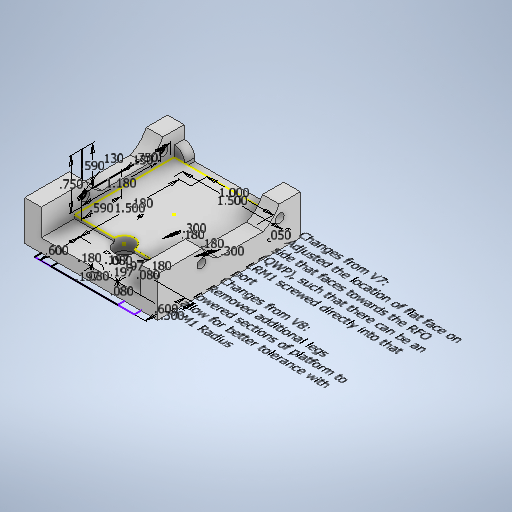
# Autodesk Inventor part: BeamsplitterMounttoPolarisPinAdapterV9
Saved by Autodesk Inventor 2025.2 (Build 292293000, 293)
## iProperties
Created: 2024-02-07
Part Number: BeamsplitterMounttoPolarisPinAdapterV9
Material: Generic
Document SubType Name: Modeling
Designer: monolithic
Density: 1 g/cm^3
Appearance: Default
Author: monolithic
Autodesk Inventor part; units mm, degrees
ref_plane "YZ Plane" through (0, 0, 0) normal (1, 0, 0) x (0, 1, 0)
ref_plane "XZ Plane" through (0, 0, 0) normal (0, 1, 0) x (-1, 0, 0)
ref_plane "XY Plane" through (0, 0, 0) normal (0, 0, 1) x (1, 0, 0)
sketch "Sketch1" plane through (0, 0, 0) normal (0, 1, 0) x (-1, 0, 0)
  line L0 (-12.7, 19.05) -> (12.7, 19.05)
  line L1 (12.7, 19.05) -> (12.7, -19.05)
  line L2 (12.7, -19.05) -> (-12.7, -19.05)
  line L3 (-12.7, -19.05) -> (-12.7, 19.05)
  line L4 (-12.7, 19.05) -> (12.7, -19.05) construction
  line L5 (12.7, 19.05) -> (-12.7, -19.05) construction
  circle A0 centre (0, 0) radius 2.286
  line L6 (12.7, 19.05) -> (-12.7, 19.05)
  line L7 (-12.7, 19.05) -> (-12.7, 34.29)
  line L8 (-12.7, 34.29) -> (12.7, 34.29)
  line L9 (12.7, 34.29) -> (12.7, 19.05)
  line L10 (-19.05, 19.05) -> (19.05, 19.05)
  line L11 (19.05, 19.05) -> (19.05, -19.05)
  line L12 (19.05, -19.05) -> (-19.05, -19.05)
  line L13 (-19.05, -19.05) -> (-19.05, 19.05)
  line L14 (-19.05, 19.05) -> (19.05, -19.05) construction
  line L15 (19.05, 19.05) -> (-19.05, -19.05) construction
  circle A1 centre (12.7, 0) radius 2.286
  circle A2 centre (-12.7, 0) radius 2.286
  line L16 (19.05, 19.05) -> (-19.05, 19.05)
  line L17 (-19.05, 19.05) -> (-19.05, 34.29)
  line L18 (-19.05, 34.29) -> (19.05, 34.29)
  line L19 (19.05, 34.29) -> (19.05, 19.05)
  circle A3 centre (0, 26.67) radius 2.286
  line L20 (-19.05, -19.05) -> (19.05, -19.05)
  line L21 (19.05, -19.05) -> (19.05, -20.32)
  line L22 (19.05, -20.32) -> (-19.05, -20.32)
  line L23 (-19.05, -20.32) -> (-19.05, -19.05)
  circle A4 centre (0, 0) radius 3.81
  circle A5 centre (-12.7, 0) radius 3.81
  circle A6 centre (12.7, 0) radius 3.81
  line L24 (0, 26.67) -> (-5.0038, 26.67)
  line L25 (-5.0038, 26.67) -> (0, 26.67)
  line L26 (0, 26.67) -> (5.0038, 26.67)
  circle A7 centre (5.0038, 26.67) radius 1.016
  circle A8 centre (-5.0038, 26.67) radius 1.016
  circle A9 centre (0, 19.05) radius 2.286
  line L27 (-19.05, 26.67) -> (19.05, 26.67)
  line L28 (0, 19.05) -> (5.004, 19.05)
  line L29 (0, 19.05) -> (-5.004, 19.05)
  circle A10 centre (5.004, 19.05) radius 1.016
  circle A11 centre (-5.004, 19.05) radius 1.016
  point P0 (12.7, 34.29)
  dimension "d0" = 38.1
  dimension "d1" = 25.4
  dimension "d2" = 4.572
  dimension "d3" = 15.24
  dimension "d4" = 38.1
  dimension "d5" = 4.572
  dimension "d6" = 4.572
  dimension "d7" = 4.572
  dimension "d10" = 1.27
  dimension "d13" = 15.24
  dimension "d14" = 7.62
  dimension "d15" = 7.62
  dimension "d16" = 7.62
  dimension "d22" = 5.0038
  dimension "d23" = 5.0038
  dimension "d24" = 2.032
  dimension "d25" = 2.032
  dimension "d28" = 4.572
  dimension "d74" = 5.004
  dimension "d75" = 5.004
  dimension "d76" = 2.032
  dimension "d77" = 2.032
  constraints: 60 end point, 12 centre point, 11 equal length, 9 coincident, 9 midpoint, 6 horizontal, 5 perpendicular, 3 point on line
  measures "d0" distance of L0.end L1.end
  measures "d1" distance of L1.end L2.end
  measures "d2" diameter of A0
  measures "d3" distance of L8.end L0.end
  measures "d4" distance of L11.end L12.end
  measures "d5" diameter of A1
  measures "d6" diameter of A2
  measures "d7" diameter of A3
  measures "d10" distance of L22.end L12.end
  measures "d13" distance of L16.end L17.end
  measures "d14" distance of point (0, 19.05) L24.start
  measures "d15" diameter of A4
  measures "d16" diameter of A5
  measures "d22" distance of L24.start L24.end
  measures "d23" distance of L24.start L26.end
  measures "d24" diameter of A7
  measures "d25" diameter of A8
  measures "d28" diameter of A9
  measures "d74" distance of L28.start L28.end
  measures "d75" distance of L28.start L29.end
  measures "d76" diameter of A10
  measures "d77" diameter of A11
extrude "Extrusion1" add sketch "Sketch1" along normal blind 6.35 contours L0 A11 | L0 A11 | A11 L0 L7 L27 A8 L24 A3 L26 A7 L9 A10 A9 | L0 A9 A10 L1 A6 L2 L3 A5 A11 | L10 L17 L27 L7 | L3 A5 L12 L13 L10 | A5 L3 A2 | L3 A2 A5 | A10 L0 | L0 A10 | A2 L3 | L3 A2 | L27 L24 A8 | L10 L11 L12 L1 A6 | L9 L27 L19 L10 | L24 L26 A3 | A6 L1 A1 | L1 A1 A6 | A7 L26 L27 | A1 L1 | L1 A1 | A0 | A4 picked at (-5.671292, 26.588952) picked at (-1.501858, 26.487641) picked at (4.336308, 26.588952)
extrude "Extrusion2" add sketch "Sketch1" along normal blind 12.7 contours L12 L2 L21 L22 L23
extrude "Extrusion3" [suppressed]
sketch "Sketch2" plane through (0, 6.35, 0) normal (0, 1, 0) x (1, 0, 0)
  circle A0 centre (0, -26.67) radius 2.286
  circle A1 centre (0, -26.67) radius 3.81
  circle A2 centre (0, -19.050315) radius 3.810006
  point P0 (0, 0)
  point P1 (0.034998, -22.860161)
  point P2 (-0.034998, -22.860161)
  dimension "d19" = 7.62
  constraints: 2 centre point, 1 coincident
  measures "d19" diameter of A1
extrude "Extrusion4" cut sketch "Sketch2" against normal blind 5.08 contours A2
sketch "Sketch3" plane through (0, 0, 0) normal (0, -1, 0) x (1, 0, 0)
  point P0 (0, 0)
extrude "Extrusion5" cut sketch "Sketch1" along normal blind 4.445 contours L0 A11 | L0 A11 | A10 L0 | L0 A10
sketch "Sketch4" plane through (19.05, 0, -20.32) normal (0, 0, -1) x (-1, 0, 0)
  point P0 (19.05, 0)
sketch "Sketch5" plane through (-19.05, 6.35, -19.05) normal (0, 0, 1) x (1, 0, 0)
  line L0 (38.1, 6.35) -> (0, 6.35) projected
  line L1 (0, 6.35) -> (10.16, 6.35)
  line L2 (10.16, 6.35) -> (10.16, 0)
  line L3 (10.16, 0) -> (0, 0)
  line L4 (0, 0) -> (0, 6.35)
  line L5 (0, 0) -> (38.1, 0) projected
  line L6 (38.1, 6.35) -> (27.94, 6.35)
  line L7 (27.94, 6.35) -> (27.94, 0)
  line L8 (27.94, 0) -> (38.1, 0)
  line L9 (38.1, 0) -> (38.1, 6.35)
  point P0 (19.05, -6.35)
  dimension "d30" = 10.16
  dimension "d31" = 10.16
  dimension "d32" = 6.35
  constraints: 16 end point, 4 parallel, 2 horizontal, 2 perpendicular, 2 point on line
  measures "d30" distance of L2.end L3.end
  measures "d31" distance of L8.end L7.end
  measures "d32" distance of L3.end L0.end
extrude "Extrusion6" cut sketch "Sketch5" against normal blind 25.4 contours L9 L5 L7 L0 | L2 L3 L4 L0
sketch "Sketch6" plane through (0, 0, 0) normal (0, -1, 0) x (1, 0, 0)
  line L0 (19.05, -20.32) -> (20.32, -20.32)
  line L1 (19.05, -20.32) -> (-19.05, -20.32) projected
  line L2 (-19.05, -20.32) -> (-20.32, -20.32)
  line L3 (-20.32, -20.32) -> (-20.32, 19.05)
  line L4 (-20.32, 19.05) -> (-19.05, 19.05)
  line L5 (-19.05, -20.32) -> (-19.05, 26.67) projected
  line L6 (20.32, -20.32) -> (20.32, 19.05)
  line L7 (20.32, 19.05) -> (19.05, 19.05)
  line L8 (19.05, 19.05) -> (19.05, -20.32)
  line L9 (-19.05, 19.05) -> (-19.05, -20.32)
  point P0 (0, 0)
  dimension "d35" = 1.27
  dimension "d36" = 1.27
  dimension "d37" = 39.37
  constraints: 16 end point, 3 horizontal, 3 point on line, 2 perpendicular, 1 collinear, 1 parallel
  measures "d35" distance of L0.start L0.end
  measures "d36" distance of L1.end L2.end
  measures "d37" distance of L2.end L3.end
extrude "Extrusion7" add sketch "Sketch6" against normal blind 15.24
sketch "Sketch7" plane through (-20.32, 0, -20.32) normal (-1, 0, 0) x (0, 0, 1)
  line L0 (46.99, 6.35) -> (39.37, 6.35) projected
  line L1 (39.37, 6.35) -> (0, 6.35) projected
  line L2 (1.27, 12.7) -> (1.27, 6.35) projected
  line L3 (1.27, 6.35) -> (20.32, 6.35)
  line L4 (20.32, 6.35) -> (35.306, 6.35)
  line L5 (35.306, 6.35) -> (35.306, 25.4)
  line L6 (35.306, 25.4) -> (35.306, 10.414)
  circle A0 centre (35.306, 10.414) radius 1.651
  line L7 (35.306, 10.414) -> (5.334, 10.414)
  circle A1 centre (5.334, 10.414) radius 1.651
  point P0 (20.32, 0)
  dimension "d40" = 19.05
  dimension "d41" = 14.986
  dimension "d42" = 19.05
  dimension "d43" = 14.986
  dimension "d44" = 3.302
  dimension "d45" = 29.972
  dimension "d46" = 3.302
  constraints: 10 end point, 3 point on line, 2 centre point, 2 coincident, 2 perpendicular
  measures "d40" distance of L2.end L3.end
  measures "d41" distance of L3.end L4.end
  measures "d42" distance of L4.end L5.end
  measures "d43" distance of L5.end L6.end
  measures "d44" diameter of A0
  measures "d45" distance of L7.start L7.end
  measures "d46" diameter of A1
extrude "Extrusion8" cut sketch "Sketch7" against normal blind 50.8
sketch "Sketch8" plane through (20.32, 0, 19.05) normal (1, 0, 0) x (0, 0, -1)
  line L0 (4.064, 10.414) -> (34.036, 10.414) projected
  line L1 (0, 15.24) -> (39.37, 15.24) projected
  line L2 (4.064, 6.35) -> (4.064, 25.4) projected
  line L3 (4.064, 10.414) -> (10.414, 10.414)
  circle A0 centre (34.036, 10.414) radius 1.651 projected
  line L4 (34.036, 10.414) -> (27.686, 10.414)
  line L5 (10.414, 10.414) -> (27.686, 10.414)
  line L6 (27.686, 10.414) -> (27.686, 15.24)
  line L7 (27.686, 15.24) -> (10.414, 15.24)
  line L8 (10.414, 15.24) -> (10.414, 10.414)
  point P0 (19.05, 0)
  dimension "d49" = 6.35
  dimension "d50" = 6.35
  constraints: 12 end point, 3 point on line, 2 parallel, 1 horizontal, 1 perpendicular
  measures "d49" distance of L3.start L3.end
  measures "d50" distance of L4.start L4.end
extrude "Extrusion9" cut sketch "Sketch8" against normal blind 50.8 contours L8 L1 L6 L0
thicken "Thicken1" operation add thickness 5.08 both sides no extend neighbours no toward (-1, 0, 0) faces at (-20.32, 3.471333, -3.302)
thicken "Thicken2" operation add thickness 5.08 both sides no extend neighbours no toward (1, 0, 0) faces at (20.32, 3.471333, -3.302)
thicken "Thicken3" operation add thickness 7.62 both sides no extend neighbours no toward (0, 0, 1) faces at (-23.283333, 7.196667, 19.05)
thicken "Thicken4" operation add thickness 7.62 both sides no extend neighbours no toward (0, 0, 1) faces at (23.283333, 7.196667, 19.05)
thicken "Thicken5" operation add thickness 2.54 both sides no extend neighbours no toward (0, 0, -1) faces at (2.963333, 2.116667, -20.32)
thicken "Thicken6" operation add thickness 5.08 both sides no extend neighbours no toward (0, 0, 1) faces at (-6.35, 2.116667, 26.67)
sketch "Sketch9" plane through (0, 0, 0) normal (0, -1, 0) x (1, 0, 0)
  line L0 (-25.4, -22.86) -> (25.4, -22.86) projected
  line L1 (25.4, -22.86) -> (25.4, 31.75) projected
  line L2 (-25.4, 31.75) -> (-25.4, -22.86) projected
  line L3 (25.4, 31.75) -> (-25.4, 31.75) projected
  line L4 (19.05, -16.637) -> (19.05, -13.335) projected
  line L5 (25.4, -22.86) -> (19.05, -22.86)
  line L6 (19.05, -22.86) -> (19.05, -16.637)
  line L7 (19.05, -16.637) -> (25.4, -16.637)
  line L8 (25.4, -16.637) -> (25.4, -22.86)
  line L9 (-19.05, 31.75) -> (-19.05, -22.86) projected
  line L10 (-25.4, -22.86) -> (-19.05, -22.86)
  line L11 (-19.05, -22.86) -> (-19.05, -16.637)
  line L12 (-19.05, -16.637) -> (-25.4, -16.637)
  line L13 (-25.4, -16.637) -> (-25.4, -22.86)
  point P0 (0, 0)
  constraints: 16 end point, 4 parallel, 2 horizontal, 2 perpendicular, 2 point on line
extrude "Extrusion10" [suppressed]
sketch "Sketch10" plane through (-25.4, 10.414, 8.636) normal (-1, 0, 0) x (0, 0, 1)
  point P0 (-8.636, -10.414)
move faces "Move1" translate (0, -1.27, 0) faces at (-21.166667, 10.414, 2.878667)
move faces "Move2" translate (0, -1.27, 0) faces at (23.283333, 10.414, 2.878667)
sketch "Sketch11" plane through (0, 6.35, 0) normal (0, 1, 0) x (1, 0, 0)
  line L0 (30.630675, 19.62998) -> (96.63484, 19.62998) construction
  line L1 (96.63484, 19.62998) -> (96.63484, -27.929905) construction
  line L2 (96.63484, -27.929905) -> (30.630675, -27.929905) construction
  line L3 (30.630675, -27.929905) -> (30.630675, 19.62998) construction
  point P0 (0, 0)
  constraints: 2 other
sketch "Sketch12" plane through (8.89, 12.7, -22.86) normal (0, 0, -1) x (-1, 0, 0)
  line L0 (27.94, -6.35) -> (17.78, -6.35) projected
  line L1 (27.94, -6.35) -> (23.876, -6.35)
  line L2 (23.876, -6.35) -> (23.876, -2.286)
  line L3 (-10.16, -6.35) -> (-10.16, 2.54) projected
  line L4 (-10.16, -6.35) -> (-6.096, -6.35)
  line L5 (0, -6.35) -> (-10.16, -6.35) projected
  line L6 (-6.096, -6.35) -> (-6.096, -2.286)
  line L7 (-6.096, -2.286) -> (-10.16, -2.286)
  arc A0 (-6.096, -6.35) -> (-10.16, -2.286) centre (-10.16, -6.35) ccw
  line L8 (23.876, -2.286) -> (27.94, -2.286)
  line L9 (27.94, -6.35) -> (27.94, 2.54) projected
  arc A1 (27.94, -2.286) -> (23.876, -6.35) centre (27.94, -6.35) ccw
  point P0 (8.89, -12.7)
  point P1 (-10.16, -2.286)
  dimension "d78" = 4.064
  dimension "d79" = 4.064
  dimension "d80" = 4.064
  dimension "d81" = 4.064
  constraints: 12 end point, 4 point on circle, 3 perpendicular, 3 tangent, 2 centre point, 2 point on line, 1 collinear, 1 horizontal
  measures "d78" distance of L0.start L1.end
  measures "d79" distance of L1.end L2.end
  measures "d80" distance of L3.start L4.end
  measures "d81" distance of L4.end L6.end
extrude "Extrusion11" add sketch "Sketch12" against normal blind 4.064 contours L0 A1 L9 | L3 A0 L4
move faces "Move3" translate (0, -6.35, 0) faces at (2.963333, 12.7, -20.32)
sketch "Sketch13" plane through (25.4, 15.24, -8.636) normal (1, 0, 0) x (0, 0, -1)
  line L0 (-17.272, 0) -> (-17.272, -6.096)
  line L1 (-17.272, 0) -> (-23.368, 0)
  line L2 (-17.272, 0) -> (-40.386, 0)
  line L3 (-17.272, 0) -> (-21.082, 0)
  arc A0 (-23.368, 0) -> (-17.272, -6.096) centre (-11.872829, 5.399171) ccw
  line L4 (0, 0) -> (6.096, 0)
  line L5 (0, 0) -> (14.224, 0)
  line L6 (0, -6.096) -> (0, 0)
  arc A1 (0, -6.096) -> (6.096, 0) centre (-5.399171, 5.399171) ccw
  point P0 (-8.636, -15.24)
  dimension "d87" = 6.096
  dimension "d88" = 3.81
  dimension "d89" = 12.7
  dimension "d90" = 6.096
  dimension "d91" = 12.7
  constraints: 6 end point, 4 point on circle, 3 point on line, 2 centre point
  measures "d87" distance of L0.start L1.end
  measures "d88" distance of L0.start L3.end
  measures "d89" radius of A0
  measures "d90" distance of L4.start L4.end
  measures "d91" radius of A1
extrude "Extrusion12" cut sketch "Sketch13" against normal blind 50.8
sketch "Sketch14" plane through (-19.05, 6.35, 31.75) normal (0, 1, 0) x (1, 0, 0)
  arc A0 (19.084998, 8.889839) -> (19.015002, 8.889839) centre (19.05, 12.699685) ccw
  arc A1 (19.084998, 8.889839) -> (19.015002, 8.889839) centre (19.05, 5.08) ccw
  line L0 (4.064, 54.61) -> (34.036, 54.61)
  line L1 (4.064, 54.61) -> (4.064, 50.546)
  line L2 (4.064, 50.546) -> (0, 50.546)
  line L3 (0, 0) -> (0, 50.546)
  line L4 (0, 0) -> (38.1, 0)
  line L5 (38.1, 0) -> (38.1, 50.546)
  line L6 (38.1, 50.546) -> (34.036, 50.546)
  line L7 (34.036, 50.546) -> (34.036, 54.61)
  line L8 (34.036, 50.546) -> (4.064, 50.546)
  line L9 (4.064, 50.546) -> (4.064, 54.61)
  line L10 (4.064, 54.61) -> (34.036, 54.61)
  line L11 (34.036, 54.61) -> (34.036, 50.546)
  circle A2 centre (19.05, 12.7) radius 2.286
  line L12 (19.05, 12.7) -> (0, 12.7)
  line L13 (0, 12.7) -> (0, 0)
  line L14 (0, 0) -> (19.05, 0)
  line L15 (19.05, 0) -> (19.05, 12.7)
  line L16 (0, 12.7) -> (38.1, 12.7)
  line L17 (38.1, 12.7) -> (38.1, 0)
  line L18 (38.1, 0) -> (0, 0)
  line L19 (0, 0) -> (0, 12.7)
  point P0 (19.05, 31.75)
  point P1 (15.239994, 12.7)
  point P2 (22.860006, 12.7)
  constraints: 24 end point, 6 parallel, 3 horizontal, 3 perpendicular
extrude "Extrusion13" cut sketch "Sketch14" against normal blind 1.27 contours A0 L16 L5 L4 L15 A1 | L15 L4 L3 L12 A0 A1 | L8 L1 L0 L7
move faces "Move4" translate (0, 0, -0.254) faces at (-18.16079, 8.891215, -18.796) (18.16079, 8.891215, -18.796)
move faces "Move5" translate (0, 0, -0.254) faces at (4.995333, 5.503333, -18.796)
sketch "Sketch15" plane through (-19.05, 6.35, 19.05) normal (0, 1, 0) x (1, 0, 0)
  line L0 (4.064, 38.1) -> (0, 38.1)
  line L1 (0, 0) -> (0, 38.1)
  line L2 (0, 0) -> (15.239994, 0)
  arc A0 (22.860006, 0) -> (15.239994, 0) centre (19.05, -0.000315) ccw
  line L3 (22.860006, 0) -> (38.1, 0)
  line L4 (38.1, 0) -> (38.1, 38.1)
  line L5 (38.1, 38.1) -> (34.036, 38.1)
  line L6 (34.036, 38.1) -> (4.064, 38.1)
  point P0 (19.05, 19.05)
body "Solid1"
